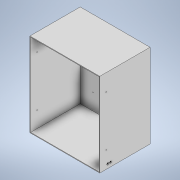
# Autodesk Inventor part: mouse_SP_shell
Saved by Autodesk Inventor 2020 (Build 240168000, 168)
## iProperties
Created: 2019-06-13
Part Number: mouse_SP_shell
Material: Generic
Document SubType Name: Modeling
Designer: Dammy
Density: 1 g/cm^3
Appearance: Default
Author: Dammy
Autodesk Inventor part; units mm, degrees
ref_plane "YZ Plane" through (0, 0, 0) normal (1, 0, 0) x (0, 1, 0)
ref_plane "XZ Plane" through (0, 0, 0) normal (0, 1, 0) x (-1, 0, 0)
ref_plane "XY Plane" through (0, 0, 0) normal (0, 0, 1) x (1, 0, 0)
sketch "Sketch2" plane through (0, 0, 0) normal (0, 0, 1) x (1, 0, 0)
  line L0 (250, -300) -> (-250, -300)
  line L1 (-250, -300) -> (-250, 300)
  line L2 (-250, 300) -> (250, 300)
  line L3 (250, 300) -> (250, -300)
  line L4 (250, -300) -> (-250, 300) construction
  line L5 (-250, -300) -> (250, 300) construction
  point P0 (0, 0)
  dimension "d0" = 500
  dimension "d1" = 600
  constraints: 12 end point, 2 midpoint, 2 parallel, 1 horizontal, 1 perpendicular
  measures "d0" distance of L1.end L2.end
  measures "d1" distance of L0.end L1.end
extrude "Base" add sketch "Sketch2" along normal blind 360
shell "Shell1" thickness 5 removed faces 1 at (-83.3333, -100, 360)
sketch "Sketch4" plane through (250, -300, 0) normal (1, 0, 0) x (0, 0, -1)
  circle A0 centre (-302.5, 28.75) radius 7.5
  line L0 (-360, 0) -> (-360, 600) projected
  line L1 (0, 0) -> (-360, 0) projected
  circle A1 centre (-282.5, 28.75) radius 7.5
  point P0 (0, 300)
  dimension "d18" = 15
  dimension "d19" = 57.5
  dimension "d20" = 28.75
  dimension "d23" = 20
  constraints: 2 centre point, 1 horizontal, 2 other
  measures "d18" diameter of A0
  measures "d19" distance from line of L0 A0.centre
  measures "d20" distance from line of L1 A0.centre
  measures "d23" distance of A0.centre A1.centre
extrude "Cable Holes" cut sketch "Sketch4" against normal up to surface (5 mm away)
sketch "Sketch5" plane through (-245, 295, 5) normal (0, 0, 1) x (1, 0, 0)
  line L0 (399.75, -474.75) -> (90.25, -474.75) construction
  line L1 (90.25, -474.75) -> (90.25, -115.25) construction
  line L2 (90.25, -115.25) -> (399.75, -115.25) construction
  line L3 (399.75, -115.25) -> (399.75, -474.75) construction
  line L4 (399.75, -474.75) -> (90.25, -115.25) construction
  line L5 (90.25, -474.75) -> (399.75, -115.25) construction
  circle A0 centre (90.25, -115.25) radius 2.75
  circle A1 centre (399.75, -115.25) radius 2.75
  circle A2 centre (90.25, -474.75) radius 2.75
  circle A3 centre (399.75, -474.75) radius 2.75
  point P0 (245, -295)
  dimension "d30" = 309.5
  dimension "d31" = 359.5
  dimension "d32" = 5.5
  dimension "d35" = 309.5
  dimension "d38" = 359.5
  constraints: 12 end point, 4 centre point, 2 horizontal, 2 midpoint, 2 parallel, 1 coincident, 1 perpendicular, 1 vertical, 6 other
  measures "d30" distance of L1.end L2.end
  measures "d31" distance of L0.end L1.end
  measures "d32" diameter of A0
  measures "d35" distance of A0.centre A1.centre
  measures "d38" distance of A0.centre A2.centre
extrude "Mount Holes inner walls" cut sketch "Sketch5" against normal up to surface (5 mm away)
sketch "Sketch6" plane through (250, -300, 0) normal (1, 0, 0) x (0, 0, -1)
  circle A0 centre (-314.25, 479.75) radius 2.625
  line L0 (-360, 595) -> (-360, 5) construction
  line L1 (-360, 595) -> (-360, 305) construction
  line L2 (-314.25, 479.75) -> (-314.25, 120.25) construction
  circle A1 centre (-314.25, 120.25) radius 2.625
  line L3 (-5, 5) -> (-5, 595) projected
  point P0 (0, 300)
  point P1 (-314.25, 300)
  point P2 (-360, 300)
  dimension "d43" = 5.25
  dimension "d44" = 359.5
  dimension "d46" = 5.25
  dimension "d63" = 309.25
  constraints: 4 end point, 2 centre point, 2 midpoint, 2 vertical, 1 coincident, 1 horizontal alignment
  measures "d43" diameter of A0
  measures "d44" distance of L2.start L2.end
  measures "d46" diameter of A1
  measures "d63" distance from line of L3 L2.start
extrude "Extrusion5" cut sketch "Sketch6" against normal up to surface (5 mm away)
mirror "Mirror2" about plane through (0, 0, 0) normal (1, 0, 0) of "Extrusion5"
sketch "Sketch7" plane through (0, 0, 0) normal (0, 0, -1) x (-1, 0, 0)
  circle A0 centre (-113.0307, -138.0307) radius 19
  circle A1 centre (-129.0307, -122.0307) radius 2.15
  line L0 (-30.7163, 0) -> (40.9179, 0) construction
  line L1 (0, 50.4838) -> (0, -80.5394) construction
  circle A2 centre (-97.0307, -122.0307) radius 2.15
  circle A3 centre (-129.0307, -154.0307) radius 2.15
  circle A4 centre (-97.0307, -154.0307) radius 2.15
  circle A5 centre (-154.75, -179.75) radius 2.75 construction
  line L2 (-154.75, -179.75) -> (-113.0307, -138.0307) construction
  line L3 (-154.75, -179.75) -> (-95.75, -179.75) construction
  line L4 (-129.0307, -122.0307) -> (-97.0307, -122.0307) construction
  line L5 (-129.0307, -154.0307) -> (-129.0307, -122.0307) construction
  point P0 (0, 0)
  point P1 (-113.0307, -122.0307)
  point P2 (-129.0307, -138.0307)
  dimension "d49" = 4.3
  dimension "d52" = 32
  dimension "d55" = 32
  dimension "d58" = 38
  dimension "d59" = 59
  dimension "d60" = 45
  constraints: 12 end point, 5 centre point, 4 horizontal, 3 equal radius, 3 vertical, 2 coincident, 2 horizontal alignment, 2 midpoint, 2 vertical alignment, 1 equal length
  measures "d49" diameter of A1
  measures "d52" distance of L4.start L4.end
  measures "d55" distance of L4.start L5.start
  measures "d58" diameter of A0
  measures "d59" distance of L2.start L2.end
  measures "d60" angle of L3 L2
extrude "Fan holes" cut sketch "Sketch7" against normal up to surface (5 mm away)
equation "\"d20\" = 0.5 * d19"
equation "\"d35\" = d30"
equation "\"d38\" = d31"
equation "\"d44\" = d31"
equation "\"d46\" = d43"
equation "\"d55\" = d52"
body "Solid1"
